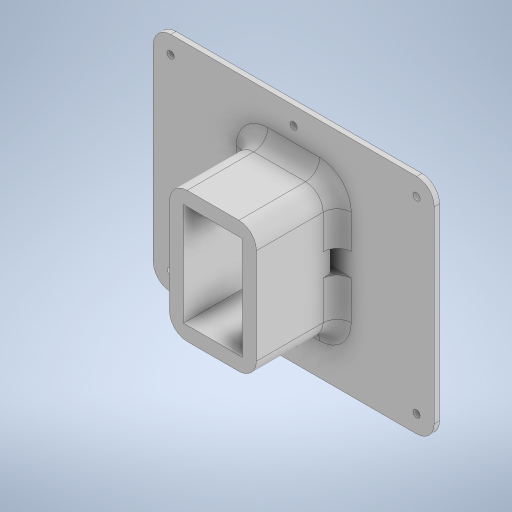
# Autodesk Inventor part: Base_Demo_1
Saved by Autodesk Inventor 2023.5 (Build 275446020, 446B)
## iProperties
Created: 2025-04-11
Part Number: Base_Demo_1
Material: Generic
Document SubType Name: Modeling
Designer: Lucky
Density: 1 g/cm^3
Appearance: Default
Author: Lucky
Autodesk Inventor part; units mm, degrees
ref_plane "YZ Plane" through (0, 0, 0) normal (1, 0, 0) x (0, 1, 0)
ref_plane "XZ Plane" through (0, 0, 0) normal (0, 1, 0) x (-1, 0, 0)
ref_plane "XY Plane" through (0, 0, 0) normal (0, 0, 1) x (1, 0, 0)
sketch "Sketch1" plane through (0, 0, 0) normal (0, 0, 1) x (1, 0, 0)
  line L0 (0, 0) -> (33.49, 0)
  line L1 (33.49, 0) -> (33.49, 58.49)
  line L2 (33.49, 58.49) -> (0, 58.49)
  line L3 (0, 58.49) -> (0, 0)
  line L4 (-8, 66.49) -> (41.49, 66.49)
  line L5 (41.49, 66.49) -> (41.49, -8)
  line L6 (41.49, -8) -> (-8, -8)
  line L7 (-8, -8) -> (-8, 66.49)
  line L8 (56.49, -8) -> (56.49, 66.49)
  line L9 (41.49, 81.49) -> (-8, 81.49)
  line L10 (-23, 66.49) -> (-23, -8)
  line L11 (-8, -23) -> (41.49, -23)
  circle A0 centre (48.99, 62.49) radius 2.55
  circle A1 centre (48.99, -4) radius 2.55
  circle A2 centre (-15.5, 62.49) radius 2.55
  circle A3 centre (-15.5, -4) radius 2.55
  arc A4 (-8, 81.49) -> (-23, 66.49) centre (-8, 66.49) ccw
  arc A5 (56.49, 66.49) -> (41.49, 81.49) centre (41.49, 66.49) ccw
  arc A6 (41.49, -23) -> (56.49, -8) centre (41.49, -8) ccw
  arc A7 (-23, -8) -> (-8, -23) centre (-8, -8) ccw
  dimension "d0" = 58.49
  dimension "d1" = 33.49
  dimension "d2" = 8
  dimension "d3" = 15
  dimension "d4" = 5.1
  dimension "d5" = 7.5
  dimension "d6" = 5.1
  dimension "d7" = 5.1
  dimension "d8" = 7.5
  dimension "d9" = 5.1
  dimension "d10" = 4
  dimension "d11" = 4
  dimension "d12" = 4
  dimension "d13" = 4
  dimension "d14" = 7.5
  dimension "d15" = 7.5
  dimension "d16" = 15
  constraints: 24 end point, 8 centre point, 8 point on circle, 8 tangent, 6 parallel, 3 equal radius, 3 perpendicular, 1 horizontal, 6 other
  measures "d0" distance between parallel lines of L0 L2
  measures "d1" distance between parallel lines of L1 L3
  measures "d2" distance between parallel lines of L2 L4
  measures "d3" distance between parallel lines of L5 L8
  measures "d4" diameter of A0
  measures "d5" distance from line of L5 A0.centre
  measures "d6" diameter of A1
  measures "d7" diameter of A2
  measures "d8" distance from line of L7 A2.centre
  measures "d9" diameter of A3
  measures "d10" distance from line of L4 A0.centre
  measures "d11" distance from line of L6 A1.centre
  measures "d12" distance from line of L4 A2.centre
  measures "d13" distance from line of L6 A3.centre
  measures "d14" distance from line of L7 A3.centre
  measures "d15" distance from line of L8 A1.centre
  measures "d16" radius of A4
extrude "Extrusion1" add sketch "Sketch1" against normal blind 46 contours L4 L5 L6 L7
fillet "Fillet1" radius 10 4 edges at (41.49, 66.49, -23) (41.49, -8, -23) (-8, 66.49, -23) (-8, -8, -23)
sketch "Sketch3" plane through (41.49, 2, 0) normal (1, 0, 0) x (0, 0, -1)
  line L0 (46, 56.49) -> (46, -2) projected
  line L1 (46, 22) -> (42, 22)
  line L2 (42, 22) -> (46, 22)
  line L3 (46, 35) -> (42, 35)
  line L4 (42, 22) -> (42, 35)
  line L5 (0, 54.49) -> (46, 54.49) projected
  line L6 (46, 65.745) -> (51, 65.745) projected
  point P0 (0, -2)
  point P1 (44, 22)
  point P2 (44, 35)
  point P3 (48.5, 65.745)
  dimension "d37" = 4
  dimension "d38" = 4
  dimension "d39" = 13
  dimension "d41" = 30.745
  constraints: 8 end point, 3 midpoint, 3 point on line, 2 horizontal
  measures "d37" distance of L3.start L3.end
  measures "d38" distance from line of L0 L1.end
  measures "d39" distance of point (44, 22) point (44, 35)
  measures "d41" vertical distance of point (48.5, 65.745) point (44, 35)
extrude "Extrusion3" cut sketch "Sketch3" against normal up to surface (8 mm away)
sketch "Sketch4" plane through (0, 0, -46) normal (0, 0, -1) x (-1, 0, 0)
  line L0 (-86.745, 92.745) -> (53.255, 92.745)
  line L1 (63.255, 82.745) -> (63.255, -24.255)
  line L2 (53.255, -34.255) -> (-86.745, -34.255)
  line L3 (-96.745, -24.255) -> (-96.745, 82.745)
  line L4 (-31.49, -8) -> (-2, -8) projected
  line L5 (-2, 66.49) -> (-31.49, 66.49) projected
  line L6 (8, 2) -> (8, 56.49) projected
  line L7 (-41.49, 56.49) -> (-41.49, 37) projected
  arc A0 (-86.745, 92.745) -> (-96.745, 82.745) centre (-86.745, 82.745) ccw
  arc A1 (63.255, 82.745) -> (53.255, 92.745) centre (53.255, 82.745) ccw
  arc A2 (53.255, -34.255) -> (63.255, -24.255) centre (53.255, -24.255) ccw
  arc A3 (-96.745, -24.255) -> (-86.745, -34.255) centre (-86.745, -24.255) ccw
  line L8 (53.255, 82.745) -> (-86.745, 82.745)
  line L9 (-86.745, 82.745) -> (-86.745, -24.255)
  line L10 (-86.745, -24.255) -> (53.255, -24.255)
  line L11 (53.255, -24.255) -> (53.255, 82.745)
  circle A4 centre (-86.745, 82.745) radius 2
  circle A5 centre (53.255, 82.745) radius 2
  circle A6 centre (53.255, -24.255) radius 2
  circle A7 centre (-86.745, -24.255) radius 2
  circle A8 centre (-16.745, 82.745) radius 2
  circle A9 centre (-16.745, -24.255) radius 2
  point P0 (0, 0)
  dimension "d46" = 160
  dimension "d47" = 127
  dimension "d48" = 74.49
  dimension "d49" = 49.49
  dimension "d50" = 55.255
  dimension "d51" = 26.255
  dimension "d52" = 10
  dimension "d53" = 10
  dimension "d54" = 107
  dimension "d55" = 140
  dimension "d56" = 4
  dimension "d57" = 4
  dimension "d58" = 4
  dimension "d59" = 4
  dimension "d60" = 4
  dimension "d61" = 4
  constraints: 16 end point, 10 centre point, 8 point on circle, 8 tangent, 4 coincident, 4 parallel, 3 equal radius, 2 midpoint, 2 perpendicular, 1 horizontal, 3 other
  measures "d46" distance between parallel lines of L1 L3
  measures "d47" distance between parallel lines of L2 L0
  measures "d48" distance between parallel lines of L4 L5
  measures "d49" distance between parallel lines of L6 L7
  measures "d50" distance between parallel lines of L1 L6
  measures "d51" distance between parallel lines of L5 L0
  measures "d52" radius of A0
  measures "d53" distance between parallel lines of L0 L8
  measures "d54" distance between parallel lines of L10 L8
  measures "d55" distance between parallel lines of L11 L9
  measures "d56" diameter of A4
  measures "d57" diameter of A5
  measures "d58" diameter of A6
  measures "d59" diameter of A7
  measures "d60" diameter of A8
  measures "d61" diameter of A9
extrude "Extrusion4" add sketch "Sketch4" along normal blind 3 contours L0 A1 L1 A2 L2 A3 L3 A0 | L8 A8 A5 L11 A6 L10 A9 A7 L9 A4
fillet "Fillet2" radius 8 9 edges at (38.5611, 63.5611, -46) (41.49, 46.745, -46) (-5.0711, 63.5611, -46) (-8, 29.245, -46) (-5.0711, -5.0711, -46) (16.745, -8, -46) (38.5611, -5.0711, -46) (41.49, 13, -46) (16.745, 66.49, -46)
body "Solid1"
